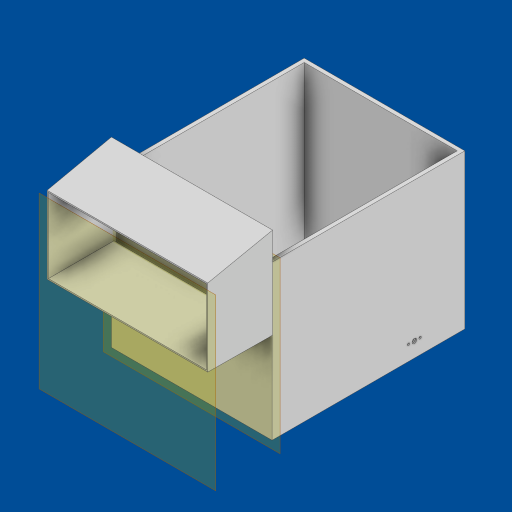
# Autodesk Inventor part: top_case
Saved by Autodesk Inventor 2023.1 (Build 271208000, 208)
## iProperties
Created: 2023-05-31
Part Number: top_case
Material: Generic
Document SubType Name: Modeling
Designer: nara atthama
Density: 1 g/cm^3
Appearance: Default
Author: nara atthama
Autodesk Inventor part; units mm, degrees
ref_plane "YZ Plane" through (0, 0, 0) normal (1, 0, 0) x (0, 1, 0)
ref_plane "XZ Plane" through (0, 0, 0) normal (0, 1, 0) x (-1, 0, 0)
ref_plane "XY Plane" through (0, 0, 0) normal (0, 0, 1) x (1, 0, 0)
sketch "Sketch1" plane through (0, 0, 0) normal (0, 1, 0) x (-1, 0, 0)
  line L0 (62.5, 75) -> (-62.5, 75)
  line L1 (-62.5, 75) -> (-62.5, -75)
  line L2 (-62.5, -75) -> (62.5, -75)
  line L3 (62.5, -75) -> (62.5, 75)
  line L4 (59.5, 72) -> (-59.5, 72)
  line L5 (-59.5, 72) -> (-59.5, -72)
  line L6 (-59.5, -72) -> (59.5, -72)
  line L7 (59.5, -72) -> (59.5, 72)
  point P0 (0, 0)
  point P1 (0, 75)
  dimension "d0" = 125
  dimension "d1" = 150
  dimension "d2" = 62.5
  dimension "d3" = 75
  dimension "d4" = 3
  constraints: 16 end point, 4 parallel, 2 perpendicular, 1 horizontal, 1 midpoint, 3 other
  measures "d0" distance of L2.end L1.end
  measures "d1" distance of L1.end L0.end
  measures "d2" distance from line of L3 point (0, 0)
  measures "d3" distance of point (0, 75) point (0, 0)
  measures "d4" distance between parallel lines of L3 L7
extrude "Extrusion1" add sketch "Sketch1" along normal blind 120
ref_plane "Work Plane3" through (62.5, 120, 75) normal (0, 0, 1) x (1, 0, 0)
sketch "Sketch3" plane through (62.5, 120, 75) normal (0, 0, 1) x (1, 0, 0)
  line L0 (-125, 21.7987) -> (0.3741, 21.7987)
  line L1 (0.3741, 21.7987) -> (0.3741, -49.0581)
  line L2 (0.3741, -49.0581) -> (-125, -49.0581)
  line L3 (-125, -49.0581) -> (-125, 21.7987)
  line L4 (-2.6259, -46.0581) -> (-2.6259, 18.7987)
  line L5 (-2.6259, 18.7987) -> (-122, 18.7987)
  line L6 (-122, 18.7987) -> (-122, -46.0581)
  line L7 (-122, -46.0581) -> (-2.6259, -46.0581)
  point P0 (-62.5, -120)
  dimension "d9" = 3
  constraints: 16 end point, 4 parallel, 2 perpendicular, 1 horizontal, 3 other
  measures "d9" distance between parallel lines of L1 L4
ref_plane "Work Plane4" through (-62.5, 0, 125) normal (0, 0, 1) x (1, 0, 0)
sketch "Sketch4" plane through (-62.5, 0, 125) normal (0, 0, 1) x (1, 0, 0)
  line L0 (3, 73.9419) -> (122.3741, 73.9419) projected
  line L1 (125.3741, 70.9419) -> (0, 70.9419) projected
  line L2 (0, 70.9419) -> (125, 70.9419)
  line L3 (125, 70.9419) -> (125, 130.9419)
  line L4 (125, 130.9419) -> (0, 130.9419)
  line L5 (0, 130.9419) -> (0, 70.9419)
  line L6 (3, 127.9419) -> (122, 127.9419)
  line L7 (122, 127.9419) -> (122, 73.9419)
  line L8 (122, 73.9419) -> (3, 73.9419)
  line L9 (3, 73.9419) -> (3, 127.9419)
  point P0 (62.5, 0)
  dimension "d11" = 3
  dimension "d12" = 60
  constraints: 16 end point, 4 parallel, 2 perpendicular, 1 horizontal, 3 other
  measures "d11" distance between parallel lines of L4 L6
  measures "d12" distance of L4.end L1.end
loft "Loft1" add profiles "Sketch3", "Sketch4" contours L0 L1 L2 L3 | L7 L6 L5 L4 / L9 L6 L7 L0 | L1 L5 L4 L3
shell "Shell1" thickness 1 removed faces 2 at (20.8333, 90.9419, 125) at (20.958, 134.5325, 75)
sketch "Sketch5" plane through (62.5, 0, 75) normal (1, 0, 0) x (0, 0, -1)
  circle A0 centre (106.1461, 11.5611) radius 0.9
  circle A1 centre (115.1461, 11.5611) radius 0.9
  circle A2 centre (110.6461, 11.5611) radius 1.75
  point P0 (75, 0)
  dimension "d18" = 9
  dimension "d19" = 1.8
  dimension "d20" = 1.8
  dimension "d21" = 4.5
  dimension "d24" = 3.5
  constraints: 3 centre point, 2 horizontal alignment, 1 coincident
  measures "d18" distance of A0.centre A1.centre
  measures "d19" diameter of A0
  measures "d20" diameter of A1
  measures "d21" distance of point (110.646, 11.561) A0.centre
  measures "d24" diameter of A2
extrude "Extrusion3" cut sketch "Sketch5" against normal through all
equation "\"d2\" = 0.5 * d0"
equation "\"d3\" = 0.5 * d1"
equation "\"d20\" = d19"
equation "\"d21\" = 0.5 * d18"
body "Solid1"
